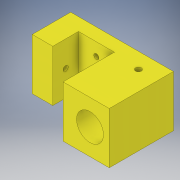
# Autodesk Inventor part: blockToSupportShaftAndPot
Saved by Autodesk Inventor 2018.2 (Build 222227000, 227)
## iProperties
Created: 2018-02-27
Part Number: blockToSupportShaftAndPot
Material: Aluminum 6061
Document SubType Name: Modeling
Designer: steele
Density: 2.7 g/cm^3
Appearance: Canary
Author: steele
Autodesk Inventor part; units mm, degrees
ref_plane "YZ Plane" through (0, 0, 0) normal (1, 0, 0) x (0, 1, 0)
ref_plane "XZ Plane" through (0, 0, 0) normal (0, 1, 0) x (-1, 0, 0)
ref_plane "XY Plane" through (0, 0, 0) normal (0, 0, 1) x (1, 0, 0)
sketch "Sketch1" plane through (0, 0, 0) normal (0, 0, 1) x (1, 0, 0)
  line L0 (-50.8, -25.4) -> (50.8, -25.4)
  line L1 (50.8, -25.4) -> (50.8, 25.4)
  line L2 (50.8, 25.4) -> (-50.8, 25.4)
  line L3 (-50.8, 25.4) -> (-50.8, -25.4)
  line L4 (-50.8, -25.4) -> (50.8, 25.4) construction
  line L5 (50.8, -25.4) -> (-50.8, 25.4) construction
  point P0 (0, 0)
  dimension "d0" = 50.8
  dimension "d1" = 101.6
  constraints: 12 end point, 2 midpoint, 2 parallel, 1 horizontal, 1 perpendicular
  measures "d0" distance of L2.end L0.start
  measures "d1" distance of L1.end L2.end
extrude "Extrusion1" add sketch "Sketch1" against normal blind 38.1
sketch "Sketch2" plane through (0, 0, 0) normal (0, 0, 1) x (1, 0, 0)
  line L0 (-50.8, 25.4) -> (50.8, 25.4) projected
  line L1 (50.8, -25.4) -> (-50.8, -25.4) projected
  line L2 (-25.4, 25.4) -> (0, 25.4)
  line L3 (0, 25.4) -> (0, -25.4)
  line L4 (0, -25.4) -> (-25.4, -25.4)
  line L5 (-25.4, -25.4) -> (-25.4, 25.4)
  line L6 (-50.8, 25.4) -> (-50.8, -25.4) projected
  point P0 (0, 0)
  dimension "d4" = 25.4
  dimension "d5" = 25.4
  constraints: 8 end point, 2 parallel, 1 horizontal, 1 midpoint, 1 perpendicular, 1 point on line
  measures "d4" distance between parallel lines of L6 L5
  measures "d5" distance between parallel lines of L5 L3
extrude "Extrusion2" cut sketch "Sketch2" against normal blind 25.4 contours L0 L3 L1 L5
sketch "Sketch3" plane through (0, 0, 0) normal (0, 0, 1) x (1, 0, 0)
  line L0 (0, 25.4) -> (0, -25.4) projected
  point P0 (0, 0)
  point P1 (31.75, 0)
  dimension "d8" = 31.75
  measures "d8" distance from line of point (31.75, 0) L0
hole "Hole1" at (31.75, 0, 0) direction (0, 0, -1) diameter 26.67 depth 31.75
sketch "Sketch4" plane through (31.75, 0, -31.75) normal (0, 0, 1) x (1, 0, 0)
  circle A0 centre (0, 0) radius 4.7625
  point P0 (-31.75, 0)
  dimension "d16" = 9.525
  constraints: 1 centre point
  measures "d16" diameter of A0
extrude "Extrusion3" cut sketch "Sketch4" against normal through all
sketch "Sketch5" plane through (-50.8, 25.4, -38.1) normal (0, 1, 0) x (1, 0, 0)
  line L0 (114.3, -38.1) -> (50.8, -38.1) construction
  line L1 (82.55, -38.1) -> (82.55, 0) construction
  line L2 (0, 0) -> (101.6, 0) construction
  line L3 (50.8, -12.7) -> (50.8, -38.1) projected
  point P0 (82.55, -15.5702)
  dimension "d19" = 15.5702
  dimension "d44" = 31.75
  constraints: 4 end point, 2 point on line, 1 midpoint, 1 vertical
  measures "d19" distance from line of L2 point (82.55, -15.57)
  measures "d44" distance between parallel lines of L1 L3
hole "Hole2" at (31.75, 25.4, -22.5298) direction (0, -1, 0) diameter 5.7912 end through all clearance for "Flat Head Machine Screw (82)" size "#12" standard "Ansi Unified Screw Threads"
sketch "Sketch6" plane through (0, 0, -38.1) normal (0, 0, -1) x (-1, 0, 0)
  line L0 (25.4, 25.4) -> (0, 25.4) construction
  line L1 (12.7, 25.4) -> (12.7, -25.4) construction
  line L2 (-50.8, -25.4) -> (50.8, -25.4) construction
  point P0 (0, 0)
  point P1 (12.7, 12.7)
  point P2 (12.7, -12.7)
  dimension "d27" = 12.7
  dimension "d28" = 12.7
  constraints: 3 point on line, 2 end point, 1 midpoint, 1 vertical
  measures "d27" distance of L1.start point (12.7, 12.7)
  measures "d28" distance from line of point (12.7, -12.7) L2
hole "Hole3" at (-12.7, 12.7, -38.1) at (-12.7, -12.7, -38.1) direction (0, 0, 1) diameter 5.1054 end through all
sketch "Sketch7" plane through (-50.8, -25.4, 0) normal (-1, 0, 0) x (0, 0, 1)
  line L0 (0, 50.8) -> (-38.1, 50.8) construction
  line L1 (-12.7, 50.8) -> (-12.7, 0) construction
  line L2 (0, 0) -> (-38.1, 0) construction
  point P0 (0, 25.4)
  point P1 (-25.4, 50.8)
  point P2 (-12.7, 25.4)
  dimension "d36" = 12.7
  constraints: 2 end point, 2 point on line, 1 midpoint, 1 vertical
  measures "d36" distance from line of point (-25.4, 50.8) L1
hole "Hole4" at (-50.8, 0, -12.7) direction (1, 0, 0) diameter 5.1054 end up to face face through (-25.4, -8.4667, -8.4667) facing (1, 0, 0) clearance for "Flat Head Machine Screw (82)" size "#10" standard "Ansi Unified Screw Threads"
sketch "Sketch8" plane through (0, 0, 0) normal (0, 0, 1) x (1, 0, 0)
  point P0 (0, 0)
sketch "Sketch9" plane through (0, 0, 0) normal (0, 0, 1) x (1, 0, 0)
  line L0 (-25.4, 25.4) -> (0, 25.4) projected
  line L1 (50.8, 25.4) -> (50.8, -25.4) projected
  line L2 (0, 25.4) -> (50.8, 25.4)
  line L3 (50.8, 25.4) -> (50.8, -25.4)
  line L4 (50.8, -25.4) -> (0, -25.4)
  line L5 (0, -25.4) -> (0, 25.4)
  circle A0 centre (31.75, 0) radius 13.335 projected
  circle A1 centre (31.75, 0) radius 13.335
  point P0 (0, 0)
  constraints: 8 end point, 2 parallel, 1 centre point, 1 coincident, 1 horizontal, 1 perpendicular
extrude "Extrusion4" add sketch "Sketch9" along normal blind 41.275
sketch "Sketch10" plane through (-50.8, 25.4, -38.1) normal (0, 1, 0) x (1, 0, 0)
  line L0 (77.7875, 0) -> (87.3125, 0) construction
  line L1 (82.55, 0) -> (82.55, -79.375) construction
  line L2 (50.8, -79.375) -> (101.6, -79.375) construction
  point P0 (50.8, -38.1)
  point P1 (82.55, -69.85)
  dimension "d47" = 9.525
  constraints: 2 end point, 2 point on line, 1 midpoint, 1 vertical
  measures "d47" distance from line of point (82.55, -69.85) L2
hole "Hole5" at (31.75, 25.4, 31.75) direction (0, -1, 0) diameter 5.7912 end through all clearance for "Flat Head Machine Screw (82)" size "#12" standard "Ansi Unified Screw Threads"
sketch "Sketch11" plane through (0, 0, -38.1) normal (0, 0, -1) x (-1, 0, 0)
  circle A0 centre (-31.75, 0) radius 4.7625 projected
  circle A1 centre (-31.75, 0) radius 6.35
  point P0 (0, 0)
  dimension "d55" = 12.7
  constraints: 1 centre point, 1 coincident
  measures "d55" diameter of A1
extrude "Extrusion5" cut sketch "Sketch11" against normal blind 3.81
sketch "Sketch13" plane through (0, 0, 41.275) normal (0, 0, 1) x (1, 0, 0)
  line L0 (50.8, -25.4) -> (-50.8, -25.4) projected
  line L1 (0, 25.4) -> (0, -25.4) projected
  line L2 (50.8, -25.4) -> (0, -25.4)
  line L3 (0, -25.4) -> (0, 25.4)
  line L4 (0, 25.4) -> (50.8, 25.4)
  line L5 (50.8, 25.4) -> (50.8, -25.4)
  point P0 (0, 0)
  constraints: 8 end point, 2 parallel, 1 horizontal, 1 perpendicular
extrude "Extrusion6" cut sketch "Sketch13" against normal blind 15.875
sketch "Sketch16" plane through (-50.8, 25.4, -38.1) normal (0, 1, 0) x (1, 0, 0)
  line L0 (25.4, -38.1) -> (0, -38.1) projected
  line L1 (25.4, -12.7) -> (20.32, -12.7)
  line L2 (20.32, -12.7) -> (20.32, -38.1)
  line L3 (20.32, -38.1) -> (25.4, -38.1)
  line L4 (25.4, -38.1) -> (25.4, -12.7)
  line L5 (50.8, -12.7) -> (50.8, -63.5) projected
  line L6 (101.6, -63.5) -> (50.8, -63.5) projected
  line L7 (50.8, -12.7) -> (55.88, -12.7)
  line L8 (55.88, -12.7) -> (55.88, -63.5)
  line L9 (55.88, -63.5) -> (50.8, -63.5)
  line L10 (50.8, -63.5) -> (50.8, -12.7)
  point P0 (50.8, -38.1)
  dimension "d60" = 5.08
  dimension "d61" = 5.08
  constraints: 16 end point, 4 parallel, 2 horizontal, 2 perpendicular, 2 point on line
  measures "d60" distance between parallel lines of L2 L4
  measures "d61" distance between parallel lines of L5 L8
extrude "Extrusion7" cut sketch "Sketch16" against normal through all
equation "\"d0\" = height"
equation "\"d1\" = width"
equation "\"d2\" = depth"
equation "\"d6\" = slotFor1x1"
equation "\"d8\" = centerOfMotorShaft"
equation "\"d9\" = shaftDiameter + clearanceForRotation"
equation "\"d44\" = centerOfMotorShaft"
equation "\"width\" = 101.6"
equation "\"height\" = 50.8"
equation "\"depth\" = 38.1"
equation "\"shaftDiameter\" = 25.4"
equation "\"centerOfMotorShaft\" = 31.75"
equation "\"clearanceForRotation\" = 1.27"
equation "\"widthOfCChannel\" = 31.75"
equation "\"slotFor1x1\" = 25.4"
body "Solid1"
